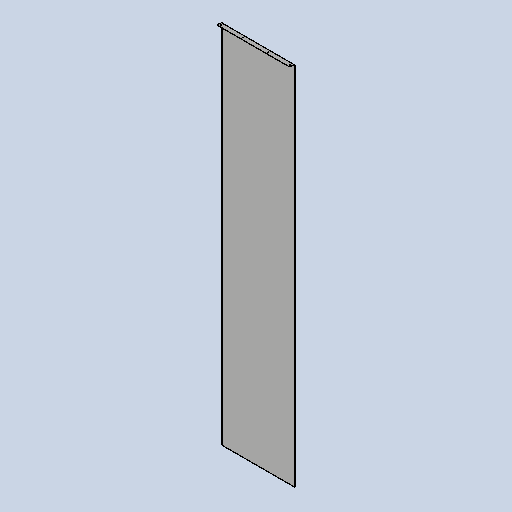
# Autodesk Inventor part: MSC 708 RIDGE 4
Saved by Autodesk Inventor 2025 (Build 290162010, 162A)
## iProperties
Created: 2024-06-20
Part Number: MSC 708 RIDGE 4
Material: Stainless Steel
Document SubType Name: Sheet Metal
Designer: pokla
Density: 8 g/cm^3
Sheet Metal Rule: AISI304 2mm Die16
Appearance: Default
Stock Number: МОО 708 пила 4
Mass: 13041.3 g
Surface Area: 16400.3 cm^2
Volume: 1630.16 cm^3
Flat Pattern Width: 40 cm
Flat Pattern Length: 203.776 cm
Flat Pattern Area: 8151.04 cm^2
Sheet Metal Width: 400,000 mm
Sheet Metal Length: 2037,761 mm
Sheet Metal Area: 815104,427 mm^2
Author: pokla
Autodesk Inventor part; units mm, degrees
ref_plane "YZ Plane" through (0, 0, 0) normal (1, 0, 0) x (0, 1, 0)
ref_plane "XZ Plane" through (0, 0, 0) normal (0, 1, 0) x (-1, 0, 0)
ref_plane "XY Plane" through (0, 0, 0) normal (0, 0, 1) x (1, 0, 0)
sketch "Sketch1" plane through (0, 0, 0) normal (0, 1, 0) x (-1, 0, 0)
  line L0 (200, 0) -> (-200, 0)
  line L1 (-200, 0) -> (-200, -2011.081)
  line L2 (-200, -2011.081) -> (200, -2011.081)
  line L3 (200, -2011.081) -> (200, 0)
  point P0 (0, 0)
  point P1 (0, 0)
  dimension "d0" = 2011.081
  dimension "d1" = 400
  measures "d0" distance of L2.end L0.start
  measures "d1" distance of L0.start L0.end
extrude "Plate1" add sketch "Sketch1" along normal blind 2
sketch "Sketch4" plane through (200, 1.8257, -1.9924) normal (0, 0.0871557, 0.9961947) x (1, 0, 0)
  line L0 (-400, 0) -> (0, 0)
  line L1 (0, 0) -> (0, 30)
  line L2 (0, 30) -> (-400, 30)
  line L3 (-400, 30) -> (-400, 0)
  constraints: 6 end point, 1 horizontal, 1 perpendicular, 1 vertical
edge flange "Flange2" height 30 angle 85 thickness 2 bend radius 2.75 thickness toward (0, 0.0871557, 0.9961947) relief straight relief width 2 relief depth 1 edges at (0, 2, 0) wall of the first edge with corners at (-200, 1.8257, -1.9924) (200, 1.8257, -1.9924) (200, -28.0602, 0.6223) (-200, -28.0602, 0.6223)
bend "Bend2"
corner "Corner2"
sketch "Sketch8" plane through (-200, -27.8858, 2.6147) normal (0, 0.0871557, 0.9961947) x (1, 0, 0)
  line L0 (400, 25.6474) -> (0, 25.6474) construction
  line L1 (0, 25.6474) -> (0, 0) projected
  line L2 (0, 0) -> (400, 0) construction
  line L3 (400, 25.6474) -> (400, 0) projected
  circle A0 centre (130, 12.8237) radius 2.5
  line L4 (200, 25.6474) -> (200, 0) construction
  circle A1 centre (270, 12.8237) radius 2.5
  circle A2 centre (390, 12.8237) radius 2.5
  circle A3 centre (10, 12.8237) radius 2.5
  point P0 (200, 28.0076)
  point P1 (200, 12.8237)
  dimension "d33" = 140
  dimension "d34" = 380
  dimension "d35" = 5
  constraints: 4 centre point, 3 equal radius, 3 midpoint, 2 end point, 2 horizontal alignment, 2 other
  measures "d33" distance of A1.centre A0.centre
  measures "d34" distance of A2.centre A3.centre
  measures "d35" diameter of A1
extrude "Cut1" cut sketch "Sketch8" against normal blind 2
fillet "Corner Round1" radius 6 2 edges at (-200, -27.973, 1.6185) (200, -27.973, 1.6185)
equation "\"d36\" = Thickness"
equation "\"d2\" = Thickness"
equation "\"d16\" = BendReliefWidth"
equation "\"d17\" = BendReliefDepth"
equation "\"d18\" = MinimumRemnant"
equation "\"d19\" = TransitionRadius"
equation "\"d22\" = BendRadius"
equation "\"d23\" = CornerReliefSize"
equation "\"d24\" = GapSize"
equation "\"d25\" = JacobiRadiusSize"
equation "\"BendReliefWidth\" = Thickness"
equation "\"BendReliefDepth\" = 0.5 * Thickness"
equation "\"CornerReliefSize\" = 4 * Thickness"
equation "\"MinimumRemnant\" = 2 * Thickness"
equation "\"TransitionRadius\" = BendRadius"
equation "\"JacobiRadiusSize\" = BendRadius"
equation "\"GapSize\" = Thickness"
equation "\"Thickness\" = 2"
equation "\"BendRadius\" = 2.75"
body "Solid1"
